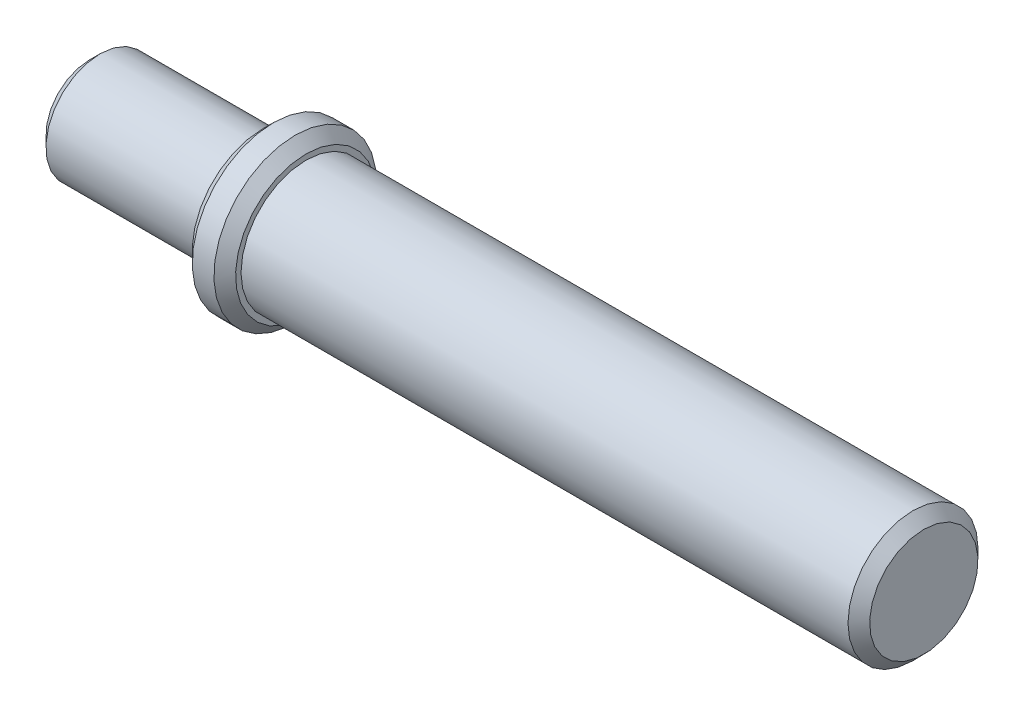
# Autodesk Inventor part: KisTenge
Saved by Autodesk Inventor 2015 (Build 190159000, 159)
## iProperties
Created: 2014-09-09
Part Number: KisTenge
Material: Generic
Document SubType Name: Modeling
Designer: laca
Density: 1 g/cm^3
Appearance: Default
Mass: 8.33255 g
Surface Area: 30.9253 cm^2
Volume: 8.33255 cm^3
Author: laca
Autodesk Inventor part; units mm, degrees
ref_plane "YZ Plane" through (0, 0, 0) normal (1, 0, 0) x (0, 1, 0)
ref_plane "XZ Plane" through (0, 0, 0) normal (0, 1, 0) x (-1, 0, 0)
ref_plane "XY Plane" through (0, 0, 0) normal (0, 0, 1) x (1, 0, 0)
sketch "Sketch1" plane through (0, 0, 0) normal (0, 0, 1) x (1, 0, 0)
  line L0 (-22.7089, -3.242) -> (-22.7089, 1.758)
  line L1 (-22.7089, 1.758) -> (-6.7089, 1.758)
  line L2 (-6.7089, 1.758) -> (-6.7089, 4.258)
  line L3 (-6.7089, 4.258) -> (-2.7089, 4.258)
  line L4 (54.2911, -3.242) -> (-22.7089, -3.242)
  line L5 (-2.7089, 2.758) -> (54.2911, 2.758)
  line L6 (54.2911, 2.758) -> (54.2911, -3.242)
  line L7 (-2.7089, 4.258) -> (-2.7089, 2.758)
  point P0 (0, 0)
  dimension "d0" = 5
  dimension "d1" = 16
  dimension "d2" = 4
  dimension "d5" = 6
  dimension "d6" = 7.5
  dimension "d7" = 57
  constraints: 16 end point, 4 perpendicular, 2 vertical, 1 horizontal
  measures "d0" distance of L0.start L0.end
  measures "d1" distance of L0.end L1.end
  measures "d2" distance of L2.end L3.end
  measures "d5" distance of L5.end L4.start
  measures "d6" distance between parallel lines of L4 L3
  measures "d7" distance of L5.start L5.end
revolve "Revolution1" add sketch "Sketch1" angle 360 about axis through (54.2911, -3.242, 0) along (-1, 0, 0)
thread "Thread1" size "M10x1.5" class "6g" standard "ANSI Metric M Profile" full length
thread "Thread2" size "M12x1.75" class "6g" standard "ANSI Metric M Profile" length 20
chamfer "Chamfer1" distance 1 angle 45 4 edges at (54.2911, -9.242, 0) (-22.7089, -8.242, 0) (-6.7089, -10.742, 0) (-2.7089, -10.742, 0)
body "Solid1"
